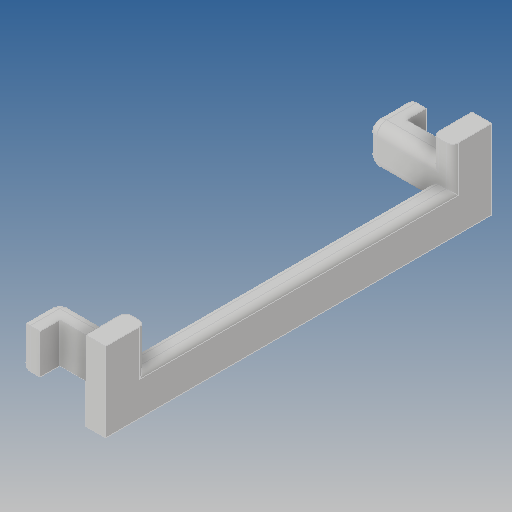
# Autodesk Inventor part: DC-DC крышка
Saved by Autodesk Inventor 2020 (Build 240168000, 168)
## iProperties
Created: 2020-03-21
Part Number: DC-DC крышка
Material: Типовые
Document SubType Name: Modeling
Designer: Iliga
Density: 1 g/cm^3
Appearance: По умолчанию
Author: Iliga
Autodesk Inventor part; units mm, degrees
ref_plane "YZ Plane" through (0, 0, 0) normal (1, 0, 0) x (0, 1, 0)
ref_plane "XZ Plane" through (0, 0, 0) normal (0, 1, 0) x (-1, 0, 0)
ref_plane "XY Plane" through (0, 0, 0) normal (0, 0, 1) x (1, 0, 0)
sketch "Эскиз1" plane through (0, 0, 0) normal (1, 0, 0) x (0, 1, 0)
  line L0 (0, 9.75) -> (4, 9.75)
  line L1 (4, 9.75) -> (4, -9.75)
  line L2 (4, -9.75) -> (0, -9.75)
  line L3 (0, -9.75) -> (0, 9.75)
  line L4 (4, 7.75) -> (3, 7.75)
  line L5 (3, 7.75) -> (3, -7.75)
  line L6 (3, -7.75) -> (4, -7.75)
  point P0 (0, 0)
  point P1 (0, 0)
  dimension "d0" = 4
  dimension "d1" = 19.5
  dimension "d2" = 2
  dimension "d3" = 1
  dimension "d4" = 2
  constraints: 14 end point, 3 perpendicular, 2 coincident, 2 horizontal, 2 parallel, 2 point on line, 1 midpoint
  measures "d0" distance between parallel lines of L1 L3
  measures "d1" distance between parallel lines of L2 L0
  measures "d2" distance between parallel lines of L0 L4
  measures "d3" distance between parallel lines of L5 L1
  measures "d4" distance between parallel lines of L2 L6
extrude "Выдавливание1" add sketch "Эскиз1" against normal blind 1
extrude "Выдавливание2" add sketch "Эскиз1" against normal blind 2 contours L1 L6 L5 L4
fillet "Сопряжение1" radius 0.5 2 edges at (-1.5, 3, -7.75) (-1.5, 3, 7.75)
sketch "Эскиз2" plane through (-1, 0, 0) normal (-1, 0, 0) x (0, 0, 1)
  line L0 (7.75, 4) -> (7.75, 3.5) projected
  line L1 (7.25, 3) -> (-7.25, 3) projected
  line L2 (-7.75, 3.5) -> (-7.75, 4) projected
  line L3 (-7.75, 4) -> (-9.75, 4) projected
  line L4 (-9.75, 4) -> (-9.75, 0) projected
  line L5 (-9.75, 0) -> (9.75, 0) projected
  line L6 (9.75, 0) -> (9.75, 4) projected
  line L7 (9.75, 4) -> (7.75, 4) projected
  line L8 (-8.75, 3) -> (-7.75, 3)
  line L9 (-8.75, 3) -> (-8.75, 1)
  line L10 (-8.75, 1) -> (-7.75, 1)
  line L11 (-7.75, 1) -> (-7.75, 3)
  arc A0 (7.25, 3) -> (7.75, 3.5) centre (7.25, 3.5) ccw projected
  arc A1 (-7.75, 3.5) -> (-7.25, 3) centre (-7.25, 3.5) ccw projected
  point P0 (0, 0)
  dimension "d10" = 1
  dimension "d11" = 1
  constraints: 8 end point, 2 vertical, 1 horizontal, 1 perpendicular
  measures "d10" distance between parallel lines of L4 L9
  measures "d11" distance between parallel lines of L5 L10
extrude "Выдавливание3" add sketch "Эскиз2" along normal blind 3.314 contours L8 L11 L10 L9
sketch "Эскиз3" plane through (-4.314, 0, 0) normal (-1, 0, 0) x (0, 0, 1)
  line L0 (-7.75, 3) -> (-8.75, 3) projected
  line L1 (-8.75, 3) -> (-8.75, 1) projected
  line L2 (-8.75, 1) -> (-7.75, 1) projected
  line L3 (-7.75, 1) -> (-7.75, 3) projected
  line L4 (-8.75, 1) -> (-9.75, 1)
  line L5 (-9.75, 1) -> (-9.75, 3)
  line L6 (-9.75, 3) -> (-8.75, 3)
  line L7 (-8.75, 3) -> (-8.75, 1)
  point P0 (0, 0)
  dimension "d15" = 1
  constraints: 8 end point, 2 parallel, 1 horizontal, 1 perpendicular
  measures "d15" distance between parallel lines of L5 L1
extrude "Выдавливание4" add sketch "Эскиз3" against normal blind 1 contours L1 L4 L5 L6
fillet "Сопряжение2" radius 0.5 6 edges at (-4.314, 2, -9.75) (-4.314, 2, -7.75) (-2.657, 3, -7.75) (-2.657, 1, -7.75) (-4.314, 3, -8.75) (-4.314, 1, -8.75)
mirror "Зеркальное отражение1" about plane through (0, 0, 0) normal (0, 0, 1) of "Выдавливание3", "Выдавливание4", "Сопряжение2"
sketch "Эскиз5" plane through (-2, 0, 0) normal (-1, 0, 0) x (0, 0, 1)
  line L0 (7.75, 4) -> (-7.75, 4) projected
  line L1 (-7.75, 4) -> (-7.75, 3.5) projected
  line L2 (-7.75, 4) -> (7.75, 4)
  line L3 (7.75, 4) -> (7.75, 2)
  line L4 (7.75, 2) -> (-7.75, 2)
  line L5 (-7.75, 2) -> (-7.75, 4)
  point P0 (0, 0)
  dimension "d23" = 2
  constraints: 8 end point, 2 parallel, 1 horizontal, 1 perpendicular, 1 point on line
  measures "d23" distance between parallel lines of L0 L4
extrude "Выдавливание6" cut sketch "Эскиз5" against normal up to surface (2 mm away)
fillet "Сопряжение4" radius 0.3 6 edges at (-1, 3.25, 7.75) (0, 3, 7.75) (0, 2, 0) (-1, 2, 0) (-1, 3.25, -7.75) (0, 3, -7.75)
